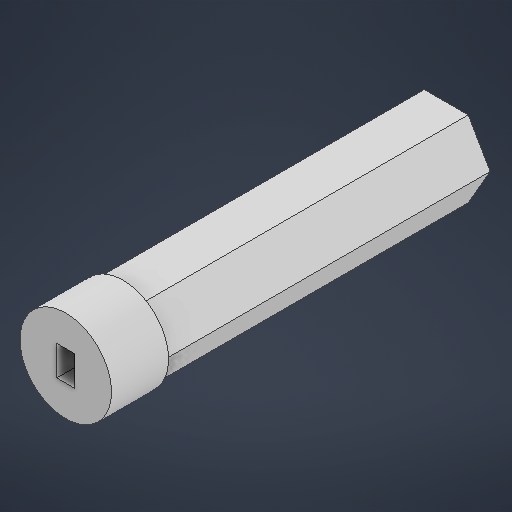
# Autodesk Inventor part: Shaft
Saved by Autodesk Inventor 2026.1 (Build 301233000, 233)
## iProperties
Created: 2025-11-03
Part Number: Shaft
Material: Generic
Document SubType Name: Modeling
Designer: randy
Density: 1 g/cm^3
Appearance: Default
Author: randy
Autodesk Inventor part; units mm, degrees
ref_plane "YZ Plane" through (0, 0, 0) normal (1, 0, 0) x (0, 1, 0)
ref_plane "XZ Plane" through (0, 0, 0) normal (0, 1, 0) x (-1, 0, 0)
ref_plane "XY Plane" through (0, 0, 0) normal (0, 0, 1) x (1, 0, 0)
sketch "Sketch1" plane through (0, 0, 0) normal (0, 0, 1) x (1, 0, 0)
  line L0 (-7.3323, 0) -> (-3.6662, 6.35)
  line L1 (-3.6662, 6.35) -> (3.6662, 6.35)
  line L2 (3.6662, 6.35) -> (7.3323, 0)
  line L3 (7.3323, 0) -> (3.6662, -6.35)
  line L4 (3.6662, -6.35) -> (-3.6662, -6.35)
  line L5 (-3.6662, -6.35) -> (-7.3323, 0)
  circle A0 centre (0, 0) radius 1.5923 construction
  dimension "d0" = 12.7
  constraints: 12 end point, 2 coincident, 1 centre point, 1 horizontal, 13 other
  measures "d0" distance between parallel lines of L4 L1
extrude "Extrusion1" add sketch "Sketch1" along normal mid plane 53.975
sketch "Sketch2" plane through (0, 0, 26.9875) normal (0, 0, 1) x (1, 0, 0)
  line L0 (3.6662, 6.35) -> (-3.6662, 6.35) projected
  line L1 (-3.6662, -6.35) -> (3.6662, -6.35) projected
  line L2 (3.6662, -6.35) -> (7.3323, 0) projected
  line L3 (7.3323, 0) -> (3.6662, 6.35) projected
  line L4 (3.6662, 6.35) -> (-3.6662, 6.35) projected
  line L5 (-3.6662, 6.35) -> (-7.3323, 0) projected
  line L6 (-7.3323, 0) -> (-3.6662, -6.35) projected
  circle A0 centre (0, 0) radius 7.62
  line L7 (1.5, -2.5) -> (-1.5, -2.5)
  line L8 (-1.5, -2.5) -> (-1.5, 2.5)
  line L9 (-1.5, 2.5) -> (1.5, 2.5)
  line L10 (1.5, 2.5) -> (1.5, -2.5)
  line L11 (1.5, -2.5) -> (-1.5, 2.5) construction
  line L12 (-1.5, -2.5) -> (1.5, 2.5) construction
  dimension "d5" = 15.24
  dimension "d6" = 3
  dimension "d7" = 5
  constraints: 12 end point, 2 midpoint, 2 parallel, 1 centre point, 1 horizontal, 1 perpendicular
  measures "d5" diameter of A0
  measures "d6" distance of L8.end L9.end
  measures "d7" distance of L7.end L8.end
extrude "Extrusion2" add sketch "Sketch2" along normal blind 9.525 contours L3 L2 L1 L6 L5 L0 | A0
sketch "Sketch3" plane through (0, 0, -26.9875) normal (0, 0, -1) x (-1, 0, 0)
  line L0 (2.54, -2.54) -> (-2.54, -2.54)
  line L1 (-2.54, -2.54) -> (-2.54, 2.54)
  line L2 (-2.54, 2.54) -> (2.54, 2.54)
  line L3 (2.54, 2.54) -> (2.54, -2.54)
  line L4 (2.54, -2.54) -> (-2.54, 2.54) construction
  line L5 (-2.54, -2.54) -> (2.54, 2.54) construction
  point P0 (0, 0)
  dimension "d11" = 5.08
  dimension "d12" = 5.08
  constraints: 12 end point, 2 midpoint, 2 parallel, 1 horizontal, 1 perpendicular
  measures "d11" distance of L1.end L2.end
  measures "d12" distance of L0.end L1.end
extrude "Extrusion3" cut sketch "Sketch3" against normal blind 3.175
fillet "Fillet1" radius 0.381 4 edges at (2.54, 0, -26.9875) (0, 2.54, -26.9875) (0, -2.54, -26.9875) (-2.54, 0, -26.9875)
body "Solid1"
